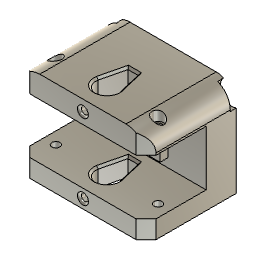
pltr_base_elegoo (Autodesk Fusion 360 design; units mm, degrees)
Autodesk Fusion 360 part; units mm, degrees
sketch "Top" plane through (0, 0, 0) normal (0, 0, 1) x (1, 0, 0)
  line L0 (0, 0) -> (-63, 0)
  line L1 (-63, 0) -> (-63, 35)
  line L2 (-63, 35) -> (0, 35)
  line L3 (0, 35) -> (0, 0)
  line L4 (-63, 12) -> (0, 12)
  line L5 (-6, 35) -> (-6, 0)
  line L6 (-57, 0) -> (-57, 35)
  line L7 (-31.5, 35) -> (-31.5, 0)
  line L8 (-63, 25) -> (0, 25)
  circle A0 centre (-31.5, 12) radius 5.5
  line L9 (-34, 25) -> (-29, 25)
  line L10 (-34, 25) -> (-36.9157, 12.9594)
  line L11 (-29, 25) -> (-26.1556, 13.2992)
  circle A1 centre (-6, 12) radius 3
  circle A2 centre (-6, 12) radius 2
  circle A3 centre (-57, 12) radius 3
  circle A4 centre (-57, 12) radius 2
  line L12 (-3.7306, 10.0378) -> (-3.166, 12.9842)
  line L13 (-3.166, 12.9842) -> (-5.4354, 14.9464)
  line L14 (-5.4354, 14.9464) -> (-8.2694, 13.9622)
  line L15 (-8.2694, 13.9622) -> (-8.834, 11.0158)
  line L16 (-8.834, 11.0158) -> (-6.5646, 9.0536)
  line L17 (-6.5646, 9.0536) -> (-3.7306, 10.0378)
  line L18 (-59.834, 12.9842) -> (-57.5646, 14.9464)
  line L19 (-57.5646, 14.9464) -> (-54.7306, 13.9622)
  line L20 (-54.7306, 13.9622) -> (-54.166, 11.0158)
  line L21 (-54.166, 11.0158) -> (-56.4354, 9.0536)
  line L22 (-56.4354, 9.0536) -> (-59.2694, 10.0378)
  line L23 (-59.2694, 10.0378) -> (-59.834, 12.9842)
  line L24 (-63, 35) -> (0, 35)
  line L25 (0, 35) -> (0, 45)
  line L26 (0, 45) -> (-63, 45)
  line L27 (-63, 45) -> (-63, 35)
  point P0 (-6, 12)
  dimension "d1" = 35
  dimension "d2" = 63
  dimension "d3" = 12
  dimension "d4" = 6
  dimension "d5" = 6
  dimension "d6" = 31.5
  dimension "d7" = 10
  dimension "d8" = 11
  dimension "d9" = 5
  dimension "d10" = 6
  dimension "d11" = 4
  dimension "d30" = 10
  constraint horizontal L0
  constraint vertical L1
  constraint horizontal L2
  constraint vertical L3
  constraint coincident L0.start L3.end
  constraint coincident L1 L4.start
  constraint coincident L3 L4.end
  constraint perpendicular L3 L4
  constraint coincident L2 L5.start
  constraint coincident L0 L5.end
  constraint perpendicular L0 L5
  constraint coincident L0 L6.start
  constraint coincident L2 L6.end
  constraint perpendicular L2 L6
  constraint coincident L2 L7.start
  constraint coincident L0 L7.end
  constraint perpendicular L0 L7
  constraint coincident L1 L8.start
  constraint coincident L3 L8.end
  constraint perpendicular L3 L8
  constraint midpoint L4 A0.centre
  constraint coincident L8 L9.start
  constraint coincident L8 L9.end
  constraint midpoint L8 L9
  constraint coincident A0 L10.end
  constraint coincident A0 L11.end
  constraint tangent A0 L11
  constraint coincident L5 P0
  constraint coincident L4 P0
  constraint concentric A1 A2
  constraint symmetric L7 A1 A3
  constraint symmetric L7 A2 A4
  constraint coincident A1 L12.start
  constraint coincident P0 A1.centre
  constraint symmetric L7 L12.start L22.end
  constraint symmetric L7 L12.end L18.start
  constraint symmetric L7 L13.end L18.end
  constraint symmetric L7 L14.end L19.end
  constraint symmetric L7 L15.end L20.end
  constraint symmetric L7 L16.end L21.end
  constraint horizontal L24
  constraint vertical L25
  constraint horizontal L26
  constraint vertical L27
  constraint collinear L3 L25
  measures "d1" distance of L0.start L2.end
  measures "d2" distance of L0.start L0.end
  measures "d3" distance of L0 L4
  measures "d4" distance of L3 L5
  measures "d5" distance of L1 L6
  measures "d6" distance of L1 L7
  measures "d7" distance of L2 L8
  measures "d8" diameter of A0
  measures "d9" distance of L9.start L9.end
  measures "d10" diameter of A1
  measures "d11" diameter of A2
  measures "d30" distance of L24 L26
extrude "Extrude1" add sketch "Top" along normal blind 47.5
sketch "Front" plane through (0, 0, 0) normal (0, 1, 0) x (1, 0, 0)
  line L0 (0, 0) -> (-73, 0)
  line L1 (0, 0) -> (0, -54.3837)
  line L2 (0, -9) -> (-63, -9)
  line L3 (0, -36.5) -> (-63, -36.5)
  line L4 (-63, -47.5) -> (0, -47.5)
  line L5 (0, 0) -> (-63, 0)
  line L6 (-31.5, 0) -> (-31.5, -47.5)
  circle A0 centre (-31.5, -42) radius 1.75
  circle A1 centre (-31.5, -4.5) radius 1.75
  line L7 (0, -32) -> (-63, -32)
  circle A2 centre (-23.75, -32) radius 3.5
  line L8 (-21.2225, -33.3946) -> (-21.2785, -30.5084)
  line L9 (-21.2785, -30.5084) -> (-23.806, -29.1138)
  line L10 (-23.806, -29.1138) -> (-26.2775, -30.6054)
  line L11 (-26.2775, -30.6054) -> (-26.2215, -33.4916)
  line L12 (-26.2215, -33.4916) -> (-23.694, -34.8862)
  line L13 (-23.694, -34.8862) -> (-21.2225, -33.3946)
  circle A3 centre (-39.25, -32) radius 3.5
  line L14 (-39.306, -34.8862) -> (-41.7775, -33.3946)
  line L15 (-36.7785, -33.4916) -> (-39.306, -34.8862)
  line L16 (-36.7225, -30.6054) -> (-36.7785, -33.4916)
  line L17 (-39.194, -29.1138) -> (-36.7225, -30.6054)
  line L18 (-41.7215, -30.5084) -> (-39.194, -29.1138)
  line L19 (-41.7775, -33.3946) -> (-41.7215, -30.5084)
  circle A4 centre (-31.5, -5) radius 3.5
  line L20 (-2, -47.5) -> (-2, 0)
  circle A5 centre (-2, -42.5) radius 6
  circle A6 centre (-61, -42.5) radius 6
  line L21 (-63, 0) -> (-63, -47.5)
  line L22 (-19, -9) -> (-19, -32)
  line L23 (-19, -23.4445) -> (-24.5, -23.4445)
  line L24 (-24.5, -23.4445) -> (-24.5, -13.4445)
  line L25 (-24.5, -13.4445) -> (-19, -13.4445)
  line L26 (-19, -13.4445) -> (-19, -23.4445)
  point P0 (-23.75, -32)
  dimension "d14" = 9
  dimension "d15" = 11
  dimension "d16" = 3.5
  dimension "d17" = 5.5
  dimension "d18" = 3.5
  dimension "d19" = 4.5
  dimension "d20" = 32
  dimension "d22" = 7.75
  dimension "d23" = 7
  dimension "d24" = 2.5
  dimension "d25" = 7
  dimension "d26" = 5
  dimension "d27" = 2
  dimension "d28" = 12
  dimension "d29" = 5
  dimension "d61" = 19
  dimension "d62" = 5.5
  dimension "d63" = 10
  constraint coincident L0.start L1.start
  constraint horizontal L0
  constraint perpendicular L0 L1
  constraint coincident L1 L2.start
  constraint perpendicular L1 L2
  constraint coincident L1 L3.start
  constraint perpendicular L1 L3
  constraint midpoint L5 L6.start
  constraint midpoint L4 L6.end
  constraint coincident L6 A0.centre
  constraint coincident L6 A1.centre
  constraint coincident L1 L7.start
  constraint perpendicular L1 L7
  constraint coincident P0 A2.centre
  constraint symmetric L6 A2 A3
  constraint symmetric L6 L8.start L14.end
  constraint symmetric L6 L8.end L18.start
  constraint symmetric L6 L9.end L17.start
  constraint symmetric L6 L10.end L16.start
  constraint symmetric L6 L11.end L15.start
  constraint symmetric L6 L12.end L14.start
  constraint coincident L6 A4.centre
  constraint coincident L4 L20.start
  constraint coincident L0 L20.end
  constraint perpendicular L0 L20
  constraint coincident L20 A5.centre
  constraint symmetric L6 A5 A6
  constraint coincident L5.end L21.start
  constraint coincident L4.start L21.end
  constraint coincident L2 L22.start
  constraint coincident L7 L22.end
  constraint perpendicular L7 L22
  constraint horizontal L23
  constraint vertical L24
  constraint horizontal L25
  constraint vertical L26
  constraint coincident L22 L23.start
  measures "d14" distance of L0 L2
  measures "d15" distance of L3 L4
  measures "d16" diameter of A0
  measures "d17" distance of L4 A0.centre
  measures "d18" diameter of A1
  measures "d19" distance of L0 A1.centre
  measures "d20" distance of L0 L7
  measures "d22" distance of L6 P0
  measures "d24" distance of P0 L13
  measures "d25" diameter of A4
  measures "d26" distance of L6.start A4.centre
  measures "d27" distance of L1 L20
  measures "d28" diameter of A5
  measures "d29" distance of L4 A5.centre
  measures "d61" distance of L1 L22
  measures "d62" distance of L23.start L23.end
  measures "d63" distance of L23.end L24.end
extrude "Extrude2" cut sketch "Front" along normal blind 30 contours L1 L2 L7 L20 | L2 L7 L20 L22 L26 | L1 L3 L7 L20 | L2 L6 L7 A2 L22 L23 L24 L25 | L3 L6 L7 A2 L20 | L2 L6 L7 A3 L21 | L22 L23 L24 L25 L26 | L3 L6 L7 A3 L21 | L7 A2 L8 L11 L12 L13 | L7 A2 L8 L9 L10 L11 | L7 A3 L16 L17 L18 L19 | L7 A3 L14 L15 L16 L19 | L7 L8 L11 L12 L13 | L7 L8 L9 L10 L11 | L7 L16 L17 L18 L19 | L7 L14 L15 L16 L19
extrude "Extrude3" cut sketch "Top" along normal blind 65 contours L4 L7 A0 | L4 L7 A0 | L4 L7 A0 | L4 L7 A0 L10 | L7 L8 A0 L9 L11 | L7 L8 A0 L9 L10
extrude "Extrude4" cut sketch "Top" along normal blind 6 from surface at 42.5 contours L5 A1 L17 | L5 A1 L17 | L4 A1 L12 | L4 A1 L12 | L4 L5 A2 L15 L16 L17 | L4 L5 A2 L12 L17 | A1 L16 | L4 L5 A2 L12 L13 L14 | A1 L13 | L6 A3 L22 | L6 A3 L22 | L4 L5 A2 | L4 L5 A2 | L4 A1 L15 | L5 A1 L14 | L5 A1 L14 | L4 L5 A2 | L4 L6 A4 L22 L23 | L4 L6 A4 L20 L21 L22 | L4 A3 L23 | A3 L21 | L4 A3 L20 | L4 A3 L20 | L4 A1 L15 | L4 L5 A2 | L4 L5 A2 L14 L15 | L4 A3 L23 | L4 L6 A4 | L4 L6 A4 | L4 L6 A4 L18 L19 L23 | L4 L6 A4 L19 L20 | L6 A3 L19 | A3 L18 | L4 L6 A4 | L4 L6 A4 | L6 A3 L19
extrude "Extrude5" cut sketch "Top" along normal blind 47.5 contours L4 L5 A2 | L4 L5 A2 | L4 L5 A2 | L4 L5 A2 | L4 L6 A4 | L4 L6 A4 | L4 L6 A4 | L4 L6 A4
extrude "Extrude6" cut sketch "Top" along normal blind 5 contours L4 L5 A2 L15 L16 L17 | L4 L5 A2 L12 L17 | L4 L5 A2 L12 L13 L14 | L4 L6 A4 L22 L23 | L4 L6 A4 L20 L21 L22 | L4 L5 A2 L14 L15 | L4 L6 A4 L18 L19 L23 | L4 L6 A4 L19 L20
chamfer "Chamfer1" distance 5 angle 45 4 edges at (0, 0, 42) (-63, 0, 42) (-63, 0, 4.5) (0, 0, 4.5)
fillet "Fillet1" radius 10 2 edges at (0, 25, 47.5) (-63, 25, 47.5)
chamfer "Chamfer2" distance 1 angle 45 8 edges at (-35.4578, 18.9797, 47.5) (-31.3264, 6.5027, 47.5) (-27.5778, 19.1496, 47.5) (-31.5, 25, 47.5) (-35.4578, 18.9797, 9) (-31.3264, 6.5027, 9) (-27.5778, 19.1496, 9) (-31.5, 25, 9)
extrude "Extrude7" cut sketch "Front" along normal blind 10 contours L6 A1 | L6 A1 | L6 A0 | L6 A0
fillet "Fillet2" radius 1 2 edges at (-33.1316, 0, 42.6328) (-33.1316, 0, 5.1328)
extrude "Extrude8" cut sketch "Front" along normal blind 35 contours L7 L8 L11 L12 L13 | L7 L8 L9 L10 L11 | L7 L16 L17 L18 L19 | L7 L14 L15 L16 L19
extrude "Extrude9" cut sketch "Front" along normal blind 10 from surface at 35 contours L7 A2 L8 L11 L12 L13 | L7 A2 L8 L9 L10 L11 | L7 A3 L16 L17 L18 L19 | L7 A3 L14 L15 L16 L19 | L7 L8 L11 L12 L13 | L7 L8 L9 L10 L11 | L7 L16 L17 L18 L19 | L7 L14 L15 L16 L19
extrude "Extrude10" cut sketch "Front" along normal blind 10 from surface at 35 contours L6 A1 A4 | L6 A1 A4 | L6 A1 | L6 A1
extrude "Extrude11" cut sketch "Front" along normal blind 5 from surface at 42 contours L1 L4 L20 A5 | L4 L20 A5 | L4 A6 L21 picked at (-60.2724, -40.4284)
extrude "Extrude12" add sketch "Front" along normal blind 4 from surface at 26 contours L22 L23 L24 L25 L26
